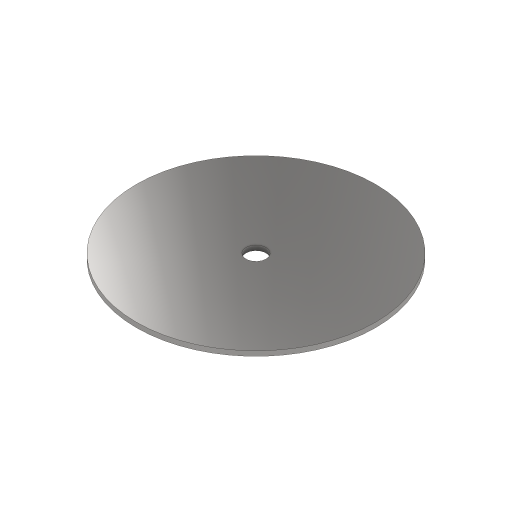
# Autodesk Inventor part: anode
Saved by Autodesk Inventor 2024.2 (Build 282272000, 272)
## iProperties
Created: 2020-09-07
Part Number: anode
Material: Stainless Steel
Document SubType Name: Modeling
Designer: mkse
Density: 8 g/cm^3
Appearance: Semi-Polished
Mass: 15.708 g
Surface Area: 40.8407 cm^2
Volume: 1.9635 cm^3
Author: mkse
Autodesk Inventor part; units mm, degrees
ref_plane "YZ Plane" through (0, 0, 0) normal (1, 0, 0) x (0, 1, 0)
ref_plane "XZ Plane" through (0, 0, 0) normal (0, 1, 0) x (-1, 0, 0)
ref_plane "XY Plane" through (0, 0, 0) normal (0, 0, 1) x (1, 0, 0)
sketch "スケッチ1" plane through (0, 0, 0) normal (0, 1, 0) x (-1, 0, 0)
  circle A0 centre (0, 0) radius 25
  dimension "d0" = 50
  constraints: 1 centre point, 1 coincident
  measures "d0" diameter of A0
extrude "押し出し1" add sketch "スケッチ1" along normal blind 1
sketch "スケッチ5" plane through (0, 0, 0) normal (0, -1, 0) x (1, 0, 0)
  circle A0 centre (0, 0) radius 2.1
  dimension "d14" = 4.2
  constraints: 1 centre point, 1 coincident
  measures "d14" diameter of A0
extrude "押し出し3" cut sketch "スケッチ5" against normal through all
